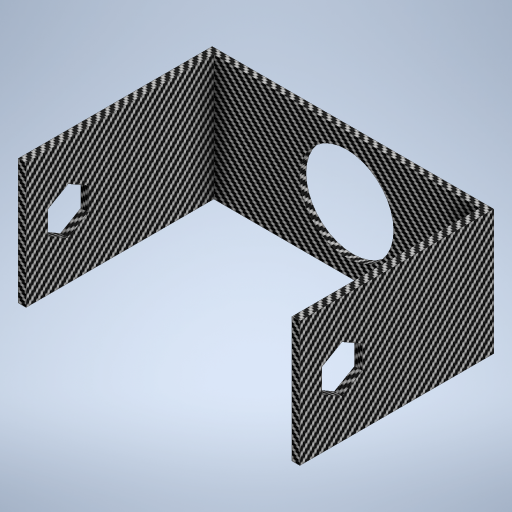
# Autodesk Inventor part: shaft to bicep
Saved by Autodesk Inventor 2023 (Build 270158000, 158)
## iProperties
Created: 2023-01-03
Part Number: shaft to bicep
Material: CFRP
Document SubType Name: Modeling
Designer: victo
Density: 1.43 g/cm^3
Appearance: Carbon Fiber
Author: victo
Autodesk Inventor part; units mm, degrees
ref_plane "YZ Plane" through (0, 0, 0) normal (1, 0, 0) x (0, 1, 0)
ref_plane "XZ Plane" through (0, 0, 0) normal (0, 1, 0) x (-1, 0, 0)
sketch "Sketch1" plane through (0, 0, 0) normal (0, 0, 1) x (1, 0, 0)
  line L0 (-3.4255, 4.1959) -> (110.8745, 4.1959)
  line L1 (110.8745, 4.1959) -> (110.8745, -46.6041)
  line L2 (110.8745, -46.6041) -> (-3.4255, -46.6041)
  line L3 (-3.4255, -46.6041) -> (-3.4255, 4.1959)
  circle A0 centre (53.7245, -21.2041) radius 19.05
  line L4 (-0.2505, 4.1959) -> (-0.2505, -46.6041)
  line L5 (107.6995, -46.6041) -> (107.6995, 4.1959)
  point P0 (0, 0)
  dimension "d0" = 114.3
  dimension "d1" = 50.8
  dimension "d2" = 38.1
  dimension "d3" = 57.15
  dimension "d4" = 25.4
  dimension "d5" = 3.175
  dimension "d6" = 3.175
  constraints: 12 end point, 4 point on line, 3 perpendicular, 2 parallel, 1 centre point, 1 horizontal
  measures "d0" distance of L1.end L2.end
  measures "d1" distance of L0.end L1.end
  measures "d2" diameter of A0
  measures "d3" distance from line of L3 A0.centre
  measures "d4" distance from line of L0 A0.centre
  measures "d5" distance between parallel lines of L4 L3
  measures "d6" distance between parallel lines of L1 L5
extrude "Extrusion1" add sketch "Sketch1" along normal blind 76.2 contours L0 L4 L2 L3 | L0 L1 L2 L5
extrude "Extrusion2" add sketch "Sketch1" against normal blind 2.54
ref_plane "Work Plane2" through (110.8745, -46.6041, 76.2) normal (1, 0, 0) x (0, 0, -1)
sketch "Sketch3" plane through (110.8745, -46.6041, 76.2) normal (1, 0, 0) x (0, 0, -1)
  line L0 (8.888, 20.6375) -> (8.888, 30.1625)
  line L1 (8.888, 30.1625) -> (17.1369, 34.925)
  line L2 (17.1369, 34.925) -> (25.3858, 30.1625)
  line L3 (25.3858, 30.1625) -> (25.3858, 20.6375)
  line L4 (25.3858, 20.6375) -> (17.1369, 15.875)
  line L5 (17.1369, 15.875) -> (8.888, 20.6375)
  line L6 (0, 0) -> (0, 50.8) projected
  line L7 (78.74, 0) -> (0, 0) projected
  point P0 (76.2, 46.6041)
  dimension "d12" = 9.525
  dimension "d13" = 9.525
  dimension "d14" = 120
  dimension "d15" = 9.525
  dimension "d16" = 120
  dimension "d17" = 9.525
  dimension "d18" = 120
  dimension "d19" = 8.888
  dimension "d20" = 15.875
  constraints: 12 end point, 3 parallel, 1 vertical
  measures "d12" distance of L0.start L0.end
  measures "d13" distance of L0.end L1.end
  measures "d14" angle of L0 L1
  measures "d15" distance of L1.end L2.end
  measures "d16" angle of L1 L2
  measures "d17" distance of L3.end L4.end
  measures "d18" angle of L3 L4
  measures "d19" distance between parallel lines of L6 L0
  measures "d20" distance from line of L7 L4.end
extrude "Extrusion3" cut sketch "Sketch3" against normal blind 127
body "Solid1"
